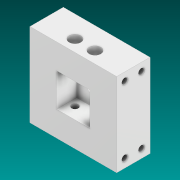
# Autodesk Inventor part: plaathouder en koppeling axis 4_5
Saved by Autodesk Inventor 2020 (Build 240168000, 168)
## iProperties
Created: 2020-05-27
Part Number: plaathouder en koppeling axis 4_5
Material: ABS Plastic
Document SubType Name: Modeling
Designer: stefa
Density: 1.06 g/cm^3
Appearance: Smooth - White
Author: stefa
Autodesk Inventor part; units mm, degrees
ref_plane "YZ Plane" through (0, 0, 0) normal (1, 0, 0) x (0, 1, 0)
ref_plane "XZ Plane" through (0, 0, 0) normal (0, 1, 0) x (-1, 0, 0)
ref_plane "XY Plane" through (0, 0, 0) normal (0, 0, 1) x (1, 0, 0)
sketch "Sketch1" plane through (0, 0, 0) normal (0, 0, 1) x (1, 0, 0)
  line L0 (-26, -25) -> (26, -25)
  line L1 (26, -25) -> (26, 25)
  line L2 (26, 25) -> (-26, 25)
  line L3 (-26, 25) -> (-26, -25)
  line L4 (-26, -25) -> (26, 25) construction
  line L5 (26, -25) -> (-26, 25) construction
  point P0 (0, 0)
  dimension "d0" = 52
  dimension "d1" = 50
  constraints: 12 end point, 2 midpoint, 2 parallel, 1 horizontal, 1 perpendicular
  measures "d0" distance of L2.end L1.end
  measures "d1" distance of L1.end L0.end
extrude "Extrusion1" add sketch "Sketch1" along normal blind 20
sketch "Sketch2" plane through (26, -25, 0) normal (1, 0, 0) x (0, 0, -1)
  circle A0 centre (-5, 5) radius 2
  line L0 (0, 0) -> (0, 50) projected
  line L1 (0, 0) -> (-20, 0) projected
  circle A1 centre (-5, 45) radius 2
  circle A2 centre (-15, 5) radius 2
  circle A3 centre (-15, 45) radius 2
  point P0 (0, 25)
  dimension "d4" = 4
  dimension "d5" = 5
  dimension "d6" = 5
  dimension "d7" = 50
  dimension "d8" = 20
  dimension "d18" = 40
  dimension "d21" = 10
  constraints: 4 centre point, 1 horizontal, 1 vertical, 6 other
  measures "d4" diameter of A0
  measures "d5" distance from line of L0 A0.centre
  measures "d6" distance from line of L1 A0.centre
  measures "d7" distance of L0.start L0.end
  measures "d8" distance of L0.start L1.end
  measures "d18" distance of A0.centre A1.centre
  measures "d21" distance of A0.centre A2.centre
hole "Hole1" at (26, -20, 15) at (26, 20, 15) at (26, 20, 5) at (26, -20, 5) direction (-1, 0, 0) diameter 3.242 depth 14 tip angle 118 countersink diameter 4 countersink angle 90 thread size "M4x0.7" class "6H" standard "ANSI Metric M Profile"
sketch "Sketch3" plane through (0, 0, 20) normal (0, 0, 1) x (1, 0, 0)
  circle A0 centre (0, 0) radius 4
  line L0 (-10, -10) -> (10, -10)
  line L1 (10, -10) -> (10, 10)
  line L2 (10, 10) -> (-10, 10)
  line L3 (-10, 10) -> (-10, -10)
  line L4 (-10, -10) -> (10, 10) construction
  line L5 (10, -10) -> (-10, 10) construction
  dimension "d31" = 8
  dimension "d32" = 20
  dimension "d33" = 20
  constraints: 12 end point, 2 midpoint, 2 parallel, 1 centre point, 1 coincident, 1 horizontal, 1 perpendicular
  measures "d31" diameter of A0
  measures "d32" distance of L1.end L2.end
  measures "d33" distance of L0.end L1.end
extrude "Extrusion2" cut sketch "Sketch3" against normal through all contours A0
extrude "Extrusion3" cut sketch "Sketch3" against normal blind 12
sketch "Sketch4" plane through (-26, -25, 0) normal (0, -1, 0) x (1, 0, 0)
  circle A0 centre (20, 13) radius 2
  line L0 (0, 0) -> (52, 0) projected
  line L1 (26, 0) -> (26, 20) construction
  circle A1 centre (20, 13) radius 3.5
  circle A2 centre (32, 13) radius 2
  circle A3 centre (32, 13) radius 3.5
  line L2 (0, 20) -> (52, 20) projected
  dimension "d38" = 4
  dimension "d40" = 6
  dimension "d42" = 7
  dimension "d48" = 7
  constraints: 4 centre point, 2 coincident, 2 end point, 2 symmetric about line, 1 midpoint, 1 vertical, 2 other
  measures "d38" diameter of A0
  measures "d40" horizontal distance of L1.start A0.centre
  measures "d42" diameter of A1
  measures "d48" distance from line of L2 A0.centre
extrude "Extrusion4" cut sketch "Sketch4" against normal blind 5
extrude "Extrusion5" cut sketch "Sketch4" against normal up to surface (15 mm away) contours A0 | A2
mirror "Mirror1" about plane through (0, 0, 0) normal (0, 1, 0) of "Extrusion4", "Extrusion5"
mirror "Mirror2" about plane through (0, 0, 0) normal (1, 0, 0) of "Hole1"
equation "\"d18\" = d7 - 2 * d6"
equation "\"d21\" = d8 - 2 * d5"
body "Solid1"
